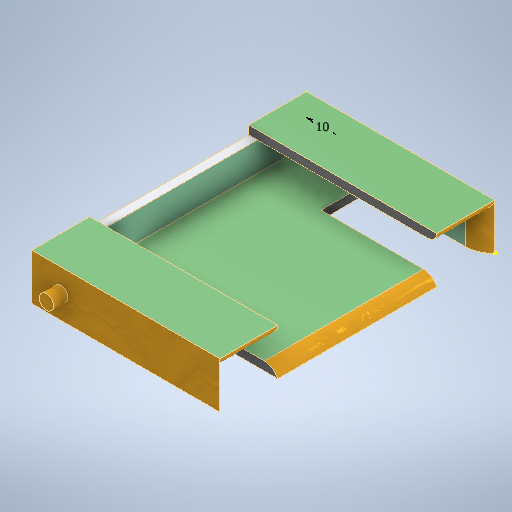
# Autodesk Inventor part: case
Saved by Autodesk Inventor 2025.1 (Build 291241020, 241B)
## iProperties
Created: 2025-01-06
Part Number: case
Material: PMMA Plastic
Document SubType Name: Modeling
Designer: User
Density: 1.188 g/cm^3
Appearance: Weld - Brass
Author: User
Autodesk Inventor part; units mm, degrees
ref_plane "YZ Plane" through (0, 0, 0) normal (1, 0, 0) x (0, 1, 0)
ref_plane "XZ Plane" through (0, 0, 0) normal (0, 1, 0) x (-1, 0, 0)
ref_plane "XY Plane" through (0, 0, 0) normal (0, 0, 1) x (1, 0, 0)
sketch "Sketch1" plane through (0, 0, 0) normal (0, 1, 0) x (-1, 0, 0)
  line L0 (0, 0) -> (65, 0)
  line L1 (65, 0) -> (65, -95)
  line L2 (65, -95) -> (0, -95)
  line L3 (0, -95) -> (0, 0)
  line L4 (65, -95) -> (0, -95)
  line L5 (0, -95) -> (0, -92)
  line L6 (0, -92) -> (65, -92)
  line L7 (65, -92) -> (65, -95)
  line L8 (65, -3) -> (0, -3)
  line L9 (65, -3) -> (0, -3)
  line L10 (0, -3) -> (0, 0)
  line L11 (0, 0) -> (65, 0)
  line L12 (65, 0) -> (65, -3)
  line L13 (65, -20) -> (0, -20)
  line L14 (0, -20) -> (0, -75)
  line L15 (0, -75) -> (65, -75)
  line L16 (65, -75) -> (65, -20)
  line L17 (40, 0) -> (40, -95)
  point P0 (40, -92)
  point P1 (40, -75)
  point P2 (40, -20)
  point P3 (40, -3)
  point P4 (0, -20)
  dimension "d0" = 95
  dimension "d1" = 65
  dimension "d4" = 3
  dimension "d7" = 65
  dimension "d8" = 3
  dimension "d13" = 55
  dimension "d14" = 20
  dimension "d24" = 25
  constraints: 36 end point, 8 parallel, 5 perpendicular, 5 point on line, 4 horizontal
  measures "d0" distance of L0.end L1.end
  measures "d1" distance of L1.end L2.end
  measures "d4" distance between parallel lines of L6 L4
  measures "d7" distance of L8.start L8.end
  measures "d8" distance between parallel lines of L11 L9
  measures "d13" distance between parallel lines of L13 L15
  measures "d14" distance between parallel lines of L15 L2
  measures "d24" distance between parallel lines of L16 L17
extrude "Extrusion1" add sketch "Sketch1" along normal blind 3
extrude "Extrusion2" add sketch "Sketch1" along normal blind 13 contours L6 L17 L2 L3 | L6 L1 L2 L17
extrude "Extrusion3" add sketch "Sketch1" along normal blind 13 contours L0 L17 L8 L3 | L0 L1 L8 L17
sketch "Sketch2" plane through (-65, 0, -95) normal (-1, 0, 0) x (0, 0, 1)
  line L0 (92, 13) -> (95, 13) projected
  line L1 (0, 0) -> (95, 0)
  line L2 (95, 0) -> (95, 13)
  line L3 (95, 13) -> (0, 13)
  line L4 (0, 13) -> (0, 0)
  constraints: 8 end point, 2 parallel, 1 horizontal, 1 perpendicular
extrude "Extrusion4" add sketch "Sketch2" against normal blind 3
sketch "Sketch3" plane through (0, 13, 0) normal (0, 1, 0) x (1, 0, 0)
  line L0 (-65, 95) -> (-65, 0) projected
  line L1 (0, 3) -> (0, 92) projected
  line L2 (-65, 0) -> (0, 0)
  line L3 (0, 0) -> (0, 20)
  line L4 (0, 20) -> (-65, 20)
  line L5 (-65, 20) -> (-65, 0)
  line L6 (-65, 95) -> (0, 95)
  line L7 (0, 95) -> (0, 75)
  line L8 (0, 75) -> (-65, 75)
  line L9 (-65, 75) -> (-65, 95)
  dimension "d15" = 20
  dimension "d16" = 20
  constraints: 16 end point, 4 parallel, 2 horizontal, 2 perpendicular, 2 point on line
  measures "d15" distance between parallel lines of L2 L4
  measures "d16" distance between parallel lines of L8 L6
extrude "Extrusion5" add sketch "Sketch3" along normal blind 3 contours L6 L7 L1 L8 L0 | L4 L1 L3 L2 L0
sketch "Sketch4" plane through (0, 0, -95) normal (0, 0, -1) x (-1, 0, 0)
  line L0 (65, 0) -> (65, 16) projected
  point P0 (0, 0)
extrude "Extrusion6" [suppressed]
extrude "Extrusion7" cut sketch "Sketch1" along normal blind 10 contours L8 L17 L13 L3 | L15 L17 L6 L3
fillet "Fillet1" radius 10 2 edges at (0, 6.5, -3) (0, 6.5, -92)
fillet "Fillet2" radius 3 2 edges at (0, 13, -10) (0, 13, -85)
fillet "Fillet3" radius 5 1 edges at (0, 3, -47.5)
sketch "Sketch5" plane through (-65, 0, 0) normal (0, 0, 1) x (1, 0, 0)
  circle A0 centre (10, 8) radius 2.5
  line L0 (0, 0) -> (0, 16) projected
  point P0 (65, 0)
  dimension "d30" = 5
  dimension "d31" = 10
  constraints: 1 centre point
  measures "d30" diameter of A0
  measures "d31" distance from line of A0.centre L0
sketch "Sketch6" plane through (-65, 0, -95) normal (0, 0, -1) x (-1, 0, 0)
  circle A0 centre (-10, 8) radius 1.0903
  line L0 (0, 0) -> (0, 16) projected
  point P0 (-65, 0)
  dimension "d32" = 10
  constraints: 1 centre point
  measures "d32" distance from line of A0.centre L0
extrude "Extrusion8" add sketch "Sketch5" along normal blind 5
body "Solid1"
